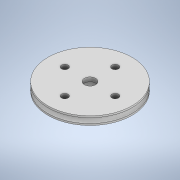
# Autodesk Inventor part: Servo_Rad
Saved by Autodesk Inventor 2021 (Build 250183000, 183)
## iProperties
Created: 2021-05-20
Part Number: Servo_Rad
Material: Generisch
Document SubType Name: Modeling
Designer: Maxim
Density: 1 g/cm^3
Appearance: Vorgabe
Author: Maxim
## iProperties of the stored document _3D-Druck.ipt
Created: 2021-06-11
Part Number: _3D-Druck
Material: Generisch
Document SubType Name: Modeling
Designer: Maxim
Density: 1 g/cm^3
Appearance: Vorgabe
Author: Maxim
Autodesk Inventor part; units mm, degrees
ref_plane "YZ Plane" through (0, 0, 0) normal (1, 0, 0) x (0, 1, 0)
ref_plane "XZ Plane" through (0, 0, 0) normal (0, 1, 0) x (-1, 0, 0)
ref_plane "XY Plane" through (0, 0, 0) normal (0, 0, 1) x (1, 0, 0)
sketch "Skizze1" plane through (0, 0, 0) normal (0, 1, 0) x (-1, 0, 0)
  circle A0 centre (0, 0) radius 10
  circle A1 centre (0, 0) radius 1.35
  dimension "d0" = 20
  dimension "d5" = 2.7
  constraints: 2 centre point, 2 coincident
  measures "d0" diameter of A0
  measures "d5" diameter of A1
extrude "Extrusion1" add sketch "Skizze1" along normal blind 2
sketch "Skizze2" plane through (0, 0, 0) normal (0, 0, 1) x (1, 0, 0)
  line L0 (-10, 0) -> (-10, 2) projected
  circle A0 centre (-10, 1) radius 0.6
  line L1 (0, -0.4) -> (0, 2.4) projected
  point P0 (0, 0)
  point P1 (-10, 1.6)
  point P2 (-10, 0.4)
  dimension "d3" = 1.2
  constraints: 1 centre point, 1 midpoint
  measures "d3" diameter of A0
revolve "Umdrehung1" add sketch "Skizze2" angle 360 about axis through (0, -10, 0) along (0, 1, 0) separate body
combine bodies "Kombinieren1" operation type subtract main body 1 bodies to subtract 2
sketch "Skizze3" plane through (0, 0, 0) normal (0, -1, 0) x (1, 0, 0)
  circle A0 centre (0, 0) radius 3.5
  circle A1 centre (0, 0) radius 2.3
  dimension "d6" = 7
  dimension "d7" = 4.6
  constraints: 2 centre point, 2 coincident
  measures "d6" diameter of A0
  measures "d7" diameter of A1
extrude "Extrusion2" add sketch "Skizze3" along normal blind 1.5 bodies 1
move faces "Verschieben1" translate (0, 1, 0) faces at (1.948, 0, -0.2912)
sketch "Skizze4" plane through (0, 2, 0) normal (0, 1, 0) x (1, 0, 0)
  circle A0 centre (0, 6) radius 0.8
  line L0 (0, 14) -> (0, -14) projected
  line L1 (14, 0) -> (-14, 0) projected
  circle A1 centre (-6, 0) radius 0.8
  circle A2 centre (0, -6) radius 0.8
  circle A3 centre (6, 0) radius 0.8
  point P0 (0, 0)
  dimension "d13" = 1.6
  dimension "d14" = 0
  dimension "d15" = 6
  dimension "d18" = 360
  constraints: 4 centre point, 9 other
  measures "d13" diameter of A0
  measures "d14" distance from line of L0 A0.centre
  measures "d15" distance from line of L1 A0.centre
extrude "Extrusion3" cut sketch "Skizze4" against normal blind 4.95 bodies 1
